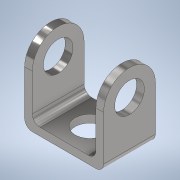
# Autodesk Inventor part: Linear Actuator Rear Mount
Saved by Autodesk Inventor 2022 (Build 260153000, 153)
## iProperties
Created: 2021-07-23
Part Number: Linear Actuator Rear Mount
Material: Generic
Document SubType Name: Modeling
Designer: John
Density: 1 g/cm^3
Appearance: Steel - Polished
Author: John
Autodesk Inventor part; units mm, degrees
ref_plane "YZ Plane" through (0, 0, 0) normal (1, 0, 0) x (0, 1, 0)
ref_plane "XZ Plane" through (0, 0, 0) normal (0, 1, 0) x (-1, 0, 0)
ref_plane "XY Plane" through (0, 0, 0) normal (0, 0, 1) x (1, 0, 0)
sketch "Sketch1" plane through (0, 0, 0) normal (0, 0, 1) x (1, 0, 0)
  line L0 (0, 0) -> (11.3, 0)
  line L1 (11.3, 0) -> (11.3, 11.2)
  line L2 (11.3, 11.2) -> (10.2, 11.2)
  line L3 (10.2, 11.2) -> (10.2, 1.1)
  line L4 (10.2, 1.1) -> (1.1, 1.1)
  line L5 (1.1, 1.1) -> (1.1, 11.2)
  line L6 (1.1, 11.2) -> (0, 11.2)
  line L7 (0, 11.2) -> (0, 0)
  dimension "d0" = 1.1
  dimension "d1" = 1.1
  dimension "d2" = 11.3
  dimension "d3" = 11.2
  constraints: 16 end point, 6 perpendicular, 2 point on line, 1 collinear, 1 horizontal
  measures "d0" distance between parallel lines of L0 L4
  measures "d1" distance of L5.end L6.end
  measures "d2" distance between parallel lines of L1 L7
  measures "d3" distance of L0.end L1.end
extrude "Extrusion1" add sketch "Sketch1" along normal blind 7.4
fillet "Fillet1" radius 3.7 4 edges at (10.75, 11.2, 7.4) (10.75, 11.2, 0) (0.55, 11.2, 7.4) (0.55, 11.2, 0)
sketch "Sketch2" plane through (11.3, 0, 7.4) normal (1, 0, 0) x (0, 0, -1)
  line L0 (7.4, 0) -> (0, 0) projected
  point P0 (3.7, 7.5)
  dimension "d14" = 7.5
  measures "d14" distance from line of L0 point (3.7, 7.5)
hole "Hole1" at (11.3, 7.5, 3.7) direction (-1, 0, 0) diameter 4.25 depth 14 tip angle 118
fillet "Fillet2" radius 1.1 4 edges at (1.1, 1.1, 3.7) (0, 0, 3.7) (11.3, 0, 3.7) (10.2, 1.1, 3.7)
sketch "Sketch3" plane through (2.2, 1.1, 0) normal (0, 1, 0) x (1, 0, 0)
  line L0 (6.9, 0) -> (0, 0) projected
  point P0 (-2.2, 0)
  point P1 (3.45, -3.7)
  point P2 (3.45, 0)
  constraints: 1 midpoint, 1 vertical alignment
hole "Hole2" at (5.65, 1.1, 3.7) direction (0, -1, 0) diameter 4.25 depth 14 tip angle 118
body "Solid1"
